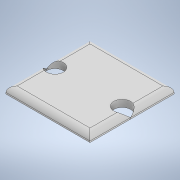
# Autodesk Inventor part: Cap
Saved by Autodesk Inventor 2020 (Build 240168000, 168)
## iProperties
Created: 2020-02-05
Part Number: Cap
Material: Generic
Document SubType Name: Modeling
Designer: maple
Density: 1 g/cm^3
Appearance: Default
Author: maple
Autodesk Inventor part; units mm, degrees
ref_plane "YZ Plane" through (0, 0, 0) normal (1, 0, 0) x (0, 1, 0)
ref_plane "XZ Plane" through (0, 0, 0) normal (0, 1, 0) x (-1, 0, 0)
ref_plane "XY Plane" through (0, 0, 0) normal (0, 0, 1) x (1, 0, 0)
sketch "Sketch1" plane through (0, 0, 0) normal (0, 1, 0) x (-1, 0, 0)
  line L0 (0, 0) -> (-15.24, 0)
  line L1 (-15.24, 0) -> (-15.24, -15.24)
  line L2 (-15.24, -15.24) -> (0, -15.24)
  line L3 (0, -15.24) -> (0, 0)
  dimension "d0" = 15.24
  dimension "d1" = 15.24
  constraints: 8 end point, 2 parallel, 1 horizontal, 1 perpendicular
  measures "d0" distance of L2.end L1.end
  measures "d1" distance of L1.end L0.end
extrude "Extrusion1" add sketch "Sketch1" along normal blind 1.27
sketch "Sketch2" plane through (0, 1.27, 0) normal (0, 1, 0) x (1, 0, 0)
  line L0 (0, 15.24) -> (0, 0) projected
  line L1 (0, 15.24) -> (1.524, 15.24)
  line L2 (1.524, 15.24) -> (1.524, 7.366)
  line L3 (1.524, 7.366) -> (0, 7.366)
  line L4 (0, 7.366) -> (0, 15.24)
  line L5 (15.24, 0) -> (15.24, 15.24) projected
  line L6 (15.24, 15.24) -> (13.716, 15.24)
  line L7 (13.716, 15.24) -> (13.716, 7.366)
  line L8 (13.716, 7.366) -> (15.24, 7.366)
  line L9 (15.24, 7.366) -> (15.24, 15.24)
  dimension "d4" = 1.524
  dimension "d5" = 7.874
  dimension "d6" = 1.524
  dimension "d7" = 7.874
  constraints: 16 end point, 4 parallel, 2 horizontal, 2 perpendicular
  measures "d4" distance of L2.end L3.end
  measures "d5" distance of L1.end L2.end
  measures "d6" distance of L8.end L7.end
  measures "d7" distance of L7.end L6.end
fillet "Fillet1" radius 1.016 4 edges at (7.62, 1.27, 0) (7.62, 1.27, -15.24) (15.24, 1.27, -7.62) (0, 1.27, -7.62)
hole "Hole2" at (1.524, 1.27, -7.366) at (13.716, 1.27, -7.366) direction (0, -1, 0) diameter 3.048 end through all
body "Solid1"
